Logo v2 (Autodesk Fusion 360 design; units mm, degrees)
Autodesk Fusion 360 part; units mm, degrees
sketch "Sketch1" plane through (0, 0, 0) normal (0, 0, 1) x (1, 0, 0)
  line L0 (27.2658, -132.272) -> (-30, -99.2094)
  line L1 (-30, -99.2094) -> (-30, -33.0822)
  line L2 (-30, -33.0822) -> (27.2658, -0.0196)
  line L3 (27.2658, -0.0196) -> (84.5305, -33.0822)
  line L4 (84.5305, -33.0822) -> (84.5305, -99.2094)
  line L5 (84.5305, -99.2094) -> (27.2658, -132.272)
  line L6 (-8.1812, -86.62) -> (27.2658, -107.0932)
  line L7 (27.2658, -107.0932) -> (62.7117, -86.62)
  line L8 (62.7117, -86.62) -> (62.7117, -45.6716)
  line L9 (62.7117, -45.6716) -> (27.2658, -25.1985)
  line L10 (27.2658, -25.1985) -> (-8.1812, -45.6716)
  line L11 (-8.1812, -45.6716) -> (-8.1812, -86.62)
  line L12 (16.2638, -72.502) -> (16.2638, -47.2612)
  line L13 (38.2046, -59.8516) -> (38.2046, -85.0914)
  line L14 (-30, -33.0822) -> (-30, -99.2094)
  line L15 (-8.1812, -86.62) -> (-8.1812, -45.6716)
  line L16 (-8.1812, -45.6716) -> (27.2658, -25.2594)
  line L17 (27.2658, -25.2594) -> (62.7117, -45.6716)
  line L18 (62.7117, -45.6716) -> (62.7117, -45.7326)
  line L19 (84.5305, -33.0822) -> (27.2658, -0.0196)
  line L20 (27.2658, -0.0196) -> (-30, -33.0822)
  line L21 (38.2046, -59.8516) -> (38.2046, -85.0914)
  line L22 (13.6721, -99.2419) -> (-8.1812, -86.62)
  line L23 (40.8862, -33.0655) -> (62.7117, -45.7326)
  line L24 (27.2658, -25.2594) -> (62.7117, -45.7326)
  line L25 (-8.1812, -86.62) -> (27.2658, -107.0932)
  line L26 (16.2638, -47.2612) -> (40.8862, -33.0655)
  line L27 (27.2658, -25.2594) -> (-8.1812, -45.6716)
  line L28 (-8.1812, -86.62) -> (-8.1812, -45.6716)
  line L29 (-8.1812, -86.62) -> (16.3868, -72.44)
  line L30 (16.3868, -72.44) -> (16.2638, -47.2612)
  line L31 (16.2638, -47.2612) -> (40.8862, -33.0655)
  line L32 (38.2046, -85.0914) -> (13.6721, -99.2419)
  line L33 (13.6721, -99.2419) -> (27.2658, -107.0932)
  line L34 (62.7117, -86.62) -> (62.7117, -45.7326)
  line L35 (27.2658, -107.0932) -> (62.7117, -86.62)
  line L36 (38.2046, -85.0914) -> (38.2046, -59.8516)
  line L37 (38.2046, -59.8516) -> (62.7117, -45.7326)
  constraint coincident L6 L22.start
  constraint coincident L9 L23.start
extrude "Extrude1" add sketch "Sketch1" along normal blind 10 contours L0 L1 L2 L3 L4 L5 L14 L19 L20 | L6 L13 L21 L22 L24 L25 L26 L29 L30 L31 L32 L36 L37 makes body 1
sketch "Sketch2" plane through (0, 0, 10) normal (0, 0, 1) x (1, 0, 0)
  line L0 (62.7117, -45.6716) -> (62.7117, -45.7326)
  line L1 (62.7117, -45.7326) -> (62.7117, -86.62)
  line L2 (62.7117, -86.62) -> (27.2658, -107.0932)
  line L3 (27.2658, -107.0932) -> (13.6721, -99.2419)
  line L4 (13.6721, -99.2419) -> (38.2046, -85.0914)
  line L5 (38.2046, -85.0914) -> (38.2046, -59.8516)
  line L6 (38.2046, -59.8516) -> (62.7117, -45.7326)
  line L7 (40.8333, -33.0959) -> (16.2638, -47.2612)
  line L8 (16.2638, -47.2612) -> (16.3868, -72.44)
  line L9 (16.3868, -72.44) -> (-8.1812, -86.62)
  line L10 (-8.1812, -86.62) -> (-8.1812, -45.6716)
  line L11 (-8.1812, -45.6716) -> (27.2658, -25.1985)
  line L12 (84.5305, -33.0822) -> (27.2658, -0.0196)
  line L13 (27.2658, -0.0196) -> (-30, -33.0822)
  line L14 (-30, -33.0822) -> (-30, -99.2094)
  line L15 (-30, -99.2094) -> (27.2658, -132.272)
  line L16 (27.2658, -132.272) -> (84.5305, -99.2094)
  line L17 (84.5305, -99.2094) -> (84.5305, -33.0822)
extrude "Extrude2" add 1 faces at (50.8941, -22.0558, 10) along direction (0, 0, 1) blind 7 separate body on bodies 1 makes body 2
sketch "Sketch3" plane through (0, 0, 17) normal (0, 0, 1) x (1, 0, 0)
  line L0 (62.7117, -45.6716) -> (62.7117, -45.7326)
  line L1 (62.7117, -45.7326) -> (62.7117, -86.62)
  line L2 (62.7117, -86.62) -> (27.2658, -107.0932)
  line L3 (27.2658, -107.0932) -> (13.6721, -99.2419)
  line L4 (13.6721, -99.2419) -> (38.2046, -85.0914)
  line L5 (38.2046, -85.0914) -> (38.2046, -59.8516)
  line L6 (38.2046, -59.8516) -> (62.7117, -45.7326)
  line L7 (40.8333, -33.0959) -> (16.2638, -47.2612)
  line L8 (16.2638, -47.2612) -> (16.3868, -72.44)
  line L9 (16.3868, -72.44) -> (-8.1812, -86.62)
  line L10 (-8.1812, -86.62) -> (-8.1812, -45.6716)
  line L11 (-8.1812, -45.6716) -> (27.2658, -25.1985)
  line L12 (84.5305, -33.0822) -> (27.2658, -0.0196)
  line L13 (27.2658, -0.0196) -> (-30, -33.0822)
  line L14 (-30, -33.0822) -> (-30, -99.2094)
  line L15 (-30, -99.2094) -> (27.2658, -132.272)
  line L16 (27.2658, -132.272) -> (84.5305, -99.2094)
  line L17 (84.5305, -99.2094) -> (84.5305, -33.0822)
  line L18 (-30, -33.0822) -> (27.2658, -0.0196)
  line L19 (84.5305, -33.0822) -> (27.2658, -0.0196)
  line L20 (-30, -33.0822) -> (-30, -99.2094)
  line L21 (-30, -99.2094) -> (27.2658, -132.272)
  line L22 (27.2658, -132.272) -> (84.5305, -99.2094)
  line L23 (84.5305, -33.0822) -> (84.5305, -99.2094)
  line L24 (-8.1812, -45.6716) -> (27.2658, -25.1985)
  line L25 (16.2638, -47.2612) -> (40.8333, -33.0959)
  line L26 (16.2638, -47.2612) -> (16.3868, -72.44)
  line L27 (-8.1812, -86.62) -> (16.3868, -72.44)
  line L28 (-8.1812, -86.62) -> (-8.1812, -45.6716)
  line L29 (62.7117, -45.6716) -> (38.2046, -59.8516)
  line L30 (38.2046, -85.0914) -> (13.6721, -99.2419)
  line L31 (27.2658, -107.0932) -> (13.6721, -99.2419)
  line L32 (27.2658, -107.0932) -> (62.7117, -86.62)
  line L33 (62.7117, -86.62) -> (62.7117, -45.6716)
  line L34 (38.2046, -85.0914) -> (38.2046, -59.8516)
  line L35 (27.2658, -25.1985) -> (40.8333, -33.0959)
  point P0 (27.2658, -25.1985)
  constraint coincident L13.end L14.start
  constraint coincident L12.end L13.start
  constraint coincident L12.start L17.end
  constraint coincident L14.end L15.start
  constraint coincident L15.end L16.start
  constraint coincident L16.end L17.start
  constraint coincident L10.end L11.start
  constraint coincident P0 L11.end
  constraint coincident L7.end L8.start
  constraint coincident L7.start L25.end
  constraint coincident L8.end L9.start
  constraint coincident L9.end L10.start
  constraint coincident L0.start L29.start
  constraint coincident L5.end L6.start
  constraint coincident L4.end L5.start
  constraint coincident L3.end L4.start
  constraint coincident L2.end L3.start
  constraint coincident L1.end L2.start
extrude "Extrude3" add sketch "Sketch3" along normal blind 5 separate body makes body 3
sketch "Sketch4" plane through (0, 0, 22) normal (0, 0, 1) x (1, 0, 0)
  line L0 (62.7117, -86.62) -> (27.2658, -107.0932)
  line L1 (27.2658, -107.0932) -> (13.6721, -99.2419)
  line L2 (13.6721, -99.2419) -> (38.2046, -85.0914)
  line L3 (38.2046, -85.0914) -> (38.2046, -59.8516)
  line L4 (38.2046, -59.8516) -> (62.7117, -45.6716)
  line L5 (62.7117, -45.6716) -> (62.7117, -86.62)
  line L6 (16.3868, -72.44) -> (-8.1812, -86.62)
  line L7 (-8.1812, -86.62) -> (-8.1812, -45.6716)
  line L8 (-8.1812, -45.6716) -> (27.2658, -25.1985)
  line L9 (27.2658, -25.1985) -> (40.8333, -33.0959)
  line L10 (40.8333, -33.0959) -> (16.2638, -47.2612)
  line L11 (16.2638, -47.2612) -> (16.3868, -72.44)
  line L12 (-30, -33.0822) -> (-30, -99.2094)
  line L13 (-30, -99.2094) -> (27.2658, -132.272)
  line L14 (27.2658, -132.272) -> (84.5305, -99.2094)
  line L15 (84.5305, -99.2094) -> (84.5305, -33.0822)
  line L16 (84.5305, -33.0822) -> (27.2658, -0.0196)
  line L17 (27.2658, -0.0196) -> (-30, -33.0822)
hidden bodies 1 2
